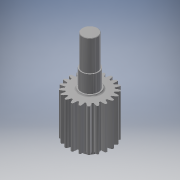
# Autodesk Inventor part: Spur Gear1
Saved by Autodesk Inventor 2018 (Build 220112000, 112)
## iProperties
Created: 2018-12-20
Part Number: Spur Gear1
Material: Steel
Document SubType Name: Modeling
Designer: Kristijan
Categories: <?xml version="1.0" encoding="UTF-16"?> <MemberInstance><Categories><FamilyTemplate><FamilyTemplateParameter ValueType="xs:double" Id="1" ObjectReferenceKey="da_z" ObjectType="kUserParameterObject"/><FamilyTemplateParameter ValueType="xs:double" Id="2" ObjectReferenceKey="da_b" ObjectType="kUserParameterObject"/><FamilyTemplateParameter ValueType="xs:double" Id="3" ObjectReferenceKey="da_beta" ObjectType="kUserParameterObject"/><FamilyTemplateParameter ValueType="xs:double" Id="4" ObjectReferenceKey="da_da" ObjectType="kUserParameterObject"/><FamilyTemplateParameter ValueType="xs:double" Id="5" ObjectReferenceKey="da_aw" ObjectType="kUserParameterObject"/><FamilyTemplateParameter ValueType="xs:string" Id="6" ObjectReferenceKey="EAIAABAAAACIAQAAAAAAAIAAAAAAAAAA" ObjectType="83910656" SubObjectId="SurfaceGeometry"/></FamilyTemplate><ParamToTemplateMap><ParamToTemplate CategoryParameter="//CategoryParameter[@InternalName='046C89C9-8512-4d59-83FE-43B91F4F132A']" TemplateParameter="1"/><ParamToTemplate CategoryParameter="//CategoryParameter[@InternalName='2552DF32-E462-4b46-AEBF-C6C7768E72AC']" TemplateParameter="2"/><ParamToTemplate CategoryParameter="//CategoryParameter[@InternalName='C9EE641D-15FC-4fae-A226-E94C4372FDD7']" TemplateParameter="3"/><ParamToTemplate><ParamToTemplate CategoryParameter="//CategoryParameter[@InternalName='00B6519A-459B-49c7-AD84-2E56D39A5744']" ConstantValue="0.000000"/></ParamToTemplate><ParamToTemplate><ParamToTemplate CategoryParameter="//CategoryParameter[@InternalName='04B31F0E-C7A6-4894-AA32-9629BEFACF47']" ConstantValue="1.000000"/></ParamToTemplate><ParamToTemplate><ParamToTemplate CategoryParameter="//CategoryParameter[@InternalName='43CBEC2E-7847-49e7-A936-2F7889FCB2D9']" ConstantValue="0.250000"/></ParamToTemplate><ParamToTemplate><ParamToTemplate CategoryParameter="//CategoryParameter[@InternalName='B1EFC894-105D-4ebd-86BF-FA20ED196853']" ConstantValue="0.350000"/></ParamToTemplate><ParamToTemplate><ParamToTemplate CategoryParameter="//CategoryParameter[@InternalName='51175063-3D10-4879-93E8-6246FE8B403D']" ConstantValue="2060000000.000000"/></ParamToTemplate><ParamToTemplate><ParamToTemplate CategoryParameter="//CategoryParameter[@InternalName='A3A52E27-4454-46a9-B0BD-C932399B70AF']" ConstantValue="0.300000"/></ParamToTemplate><ParamToTemplate><ParamToTemplate CategoryParameter="//CategoryParameter[@InternalName='91B76062-C214-41d9-B1B9-14D2AB99603D']" ConstantValue="0.500000"/></ParamToTemplate><ParamToTemplate><ParamToTemplate CategoryParameter="//CategoryParameter[@InternalName='374E806E-8B8A-4dda-A9AA-1039D6500AD2']" ConstantValue="2.000000"/></ParamToTemplate><ParamToTemplate><ParamToTemplate CategoryParameter="//CategoryParameter[@InternalName='2D373A89-B862-43d6-8D0B-0CBF12AB9F6C']" ConstantValue="0.349066"/></ParamToTemplate><ParamToTemplate CategoryParameter="//CategoryParameter[@InternalName='37777632-D6A2-4fac-9D53-DB8ACD95C989']" TemplateParameter="4"/><ParamToTemplate CategoryParameter="//CategoryParameter[@InternalName='FD1017F1-B727-4f7e-9707-0F86F1FF9423']" TemplateParameter="5"/><ParamToTemplate><ParamToTemplate CategoryParameter="//CategoryParameter[@InternalName='9E1B4470-B2D3-4ff1-B813-535BB4CDF51A']" ConstantValue="3520000.000000"/></ParamToTemplate><ParamToTemplate><ParamToTemplate CategoryParameter="//CategoryParameter[@InternalName='F8452263-BFF6-458c-9FB1-07C4B99E95CD']" ConstantValue="11400000.000000"/></ParamToTemplate><ParamToTemplate><ParamToTemplate CategoryParameter="//CategoryParameter[@InternalName='3E3BB259-FD49-497f-8171-6EBC954A3479']" ConstantValue="2.000000"/></ParamToTemplate><ParamToTemplate CategoryParameter="//CategoryParameter[@InternalName='27C3BAF2-7550-4e4b-AE2C-0DB134B7D9B7']" TemplateParameter="6"/></ParamToTemplateMap><Category DisplayName="Gear" InternalName="DC85795E-93AB-48d5-8EEE-5A27447B64BD" Mnemonic="Gear"><CategoryParameter DisplayName="z" InternalName="046C89C9-8512-4d59-83FE-43B91F4F132A" Mnemonic="z"/><CategoryParameter DisplayName="b" InternalName="2552DF32-E462-4b46-AEBF-C6C7768E72AC" Mnemonic="b"/><CategoryParameter DisplayName="||b|" InternalName="C9EE641D-15FC-4fae-A226-E94C4372FDD7" Mnemonic="beta"/><CategoryParameter DisplayName="x" InternalName="00B6519A-459B-49c7-AD84-2E56D39A5744" Mnemonic="x"/><CategoryParameter DisplayName="a*" InternalName="04B31F0E-C7A6-4894-AA32-9629BEFACF47" Mnemonic="a"/><CategoryParameter DisplayName="c*" InternalName="43CBEC2E-7847-49e7-A936-2F7889FCB2D9" Mnemonic="c"/><CategoryParameter DisplayName="r|.f|*" InternalName="B1EFC894-105D-4ebd-86BF-FA20ED196853" Mnemonic="rf"/><CategoryParameter DisplayName="E" InternalName="51175063-3D10-4879-93E8-6246FE8B403D" Mnemonic="E"/><CategoryParameter DisplayName="||m|" InternalName="A3A52E27-4454-46a9-B0BD-C932399B70AF" Mnemonic="mi"/><Category DisplayName="SpurGear" InternalName="26C5A22E-A91E-4dfd-A3B3-23CCAFAE1764" Mnemonic="SpurGear"><CategoryParameter DisplayName="m" InternalName="91B76062-C214-41d9-B1B9-14D2AB99603D" Mnemonic="m"/><CategoryParameter DisplayName="P" InternalName="374E806E-8B8A-4dda-A9AA-1039D6500AD2" Mnemonic="PP"/><CategoryParameter DisplayName="||a|" InternalName="2D373A89-B862-43d6-8D0B-0CBF12AB9F6C" Mnemonic="alpha"/><CategoryParameter DisplayName="d|.a|" InternalName="37777632-D6A2-4fac-9D53-DB8ACD95C989" Mnemonic="da"/><CategoryParameter DisplayName="a|.w|" InternalName="FD1017F1-B727-4f7e-9707-0F86F1FF9423" Mnemonic="aw"/><CategoryParameter DisplayName="||s||.Flim|" InternalName="9E1B4470-B2D3-4ff1-B813-535BB4CDF51A" Mnemonic="sFlim"/><CategoryParameter DisplayName="||s||.Hlim|" InternalName="F8452263-BFF6-458c-9FB1-07C4B99E95CD" Mnemonic="sHlim"/><CategoryParameter DisplayName="type" InternalName="3E3BB259-FD49-497f-8171-6EBC954A3479" Mnemonic="type"/><CategoryParameter DisplayName="PitchDiameter" InternalName="27C3BAF2-7550-4e4b-AE2C-0DB134B7D9B7" Mnemonic="IDS_PITCHDIAM"/></Category></Category></Categories></MemberInstance>
Density: 1 g/cm^3
Appearance: Steel
CustomPartVersion: 1
Author: Kristijan
Autodesk Inventor part; units mm, degrees
sketch "Sketch1" plane through (0, 0, 0) normal (0, 0, 1) x (1, 0, 0)
  circle A0 centre (0, 0) radius 57.5
  dimension "d0" = 115
  constraints: 1 centre point
  measures "d0" diameter of A0
extrude "Extrusion1" add sketch "Sketch1" along normal blind 110
ref_plane "Work Plane2" through (0, 0, 55) normal (0, 0, 1) x (1, 0, 0)
sketch "Sketch2" plane through (0, 0, 0) normal (0, 0, -1) x (-1, 0, 0)
  circle A0 centre (0, 0) radius 57.5 projected
  circle A1 centre (0, 0) radius 52.5
  dimension "d3" = 105
  constraints: 1 centre point, 1 coincident
  measures "d3" diameter of A1
surface extrude "Pitch Diameter" sketch "Sketch2" against normal through all shown no curves A1
ref_plane "Work Plane8" through (0, 0, 0) normal (0.9888308, 0.1490423, 0) x (0, 0, 1)
ref_plane "Work Plane9" through (0, 0, 0) normal (1, 0, 0) x (0, 1, 0)
spur gear teeth "Spur Gear" teeth 21 pitch diameter 105 tip diameter 115 root diameter 92.5 face width 110 start plane through (0, 0, 0) normal (0, 0, -1) x (-1, 0, 0)
sketch "Sketch3" plane through (0, 0, 110) normal (0, 0, 1) x (1, 0, 0)
  point P0 (0, 0)
sketch "Sketch4" plane through (0, 0, 0) normal (1, 0, 0) x (0, 1, 0)
  line L0 (0, 110) -> (29, 110)
  line L1 (25.4645, 113.5355) -> (22.5, 113.5355)
  line L2 (22.5, 113.5355) -> (22.5, 158.5355)
  line L3 (22.5, 158.5355) -> (20, 158.5355)
  line L4 (20, 158.5355) -> (20, 237.5355)
  line L5 (19, 238.5355) -> (0, 238.5355)
  line L6 (0, 238.5355) -> (0, 110)
  line L7 (19, 238.5355) -> (20, 237.5355)
  arc A0 (25.4645, 113.5355) -> (29, 110) centre (30.2941, 114.8296) ccw
  point P0 (0, 0)
  point P1 (20, 238.5355)
  point P2 (57.4598, 0)
  point P3 (34.1447, 0)
  dimension "d49" = 29
  dimension "d50" = 5
  dimension "d52" = 22.5
  dimension "d53" = 20
  dimension "d54" = 80
  dimension "d55" = 1
  dimension "d56" = 45
  dimension "d86" = 45
  constraints: 16 end point, 4 perpendicular, 2 horizontal, 2 point on circle, 2 point on line, 1 centre point
  measures "d49" distance of L0.start L0.end
  measures "d50" distance of L0.end L1.start
  measures "d52" distance between parallel lines of L6 L2
  measures "d53" distance between parallel lines of L6 L4
  measures "d54" distance of L3.end point (20, 238.536)
  measures "d55" distance of L5.start point (20, 238.536)
  measures "d56" angle of L5 L7
  measures "d86" distance of L1.end L2.end
revolve "Revolution1" add sketch "Sketch4" angle 360 about axis through (0, 0, 238.5355) along (0, 0, -1)
sketch "Sketch5" plane through (0, 0, 0) normal (1, 0, 0) x (0, 1, 0)
  line L0 (0, 0) -> (24, 0)
  line L1 (24, -5) -> (24, -5)
  line L2 (24, -5) -> (22.5, -5)
  line L3 (22.5, -5) -> (22.5, -24)
  line L4 (21.5, -25) -> (0, -25)
  line L5 (0, -25) -> (0, 0)
  line L6 (35.0562, 0) -> (46.2644, 0) projected
  line L7 (45.4437, 0) -> (45.4437, 110) construction
  line L8 (34.1447, 0) -> (37.5065, 0) construction
  line L9 (45.4437, 0) -> (29, 0) construction
  arc A0 (29, 0) -> (24, -5) centre (29, -5) ccw
  line L10 (22.5, -24) -> (21.5, -25)
  line L11 (24, 0) -> (29, 0)
  line L12 (24.6065, 0) -> (34.1447, 0) projected
  line L13 (0, -78) -> (0, 293) projected
  point P0 (22.5, -25)
  dimension "d73" = 5
  dimension "d74" = 22.5
  dimension "d75" = 20
  dimension "d76" = 1.5
  dimension "d77" = 1
  dimension "d78" = 45
  dimension "d79" = 25
  constraints: 18 end point, 5 perpendicular, 4 point on line, 3 tangent, 2 horizontal, 2 point on circle, 1 centre point, 1 collinear
  measures "d73" radius of A0
  measures "d74" distance of point (22.5, -25) L4.end
  measures "d75" distance of L2.end point (22.5, -25)
  measures "d76" distance of L1.end L2.end
  measures "d77" distance of L3.end point (22.5, -25)
  measures "d78" angle of L3 L10
  measures "d79" distance of L4.end L0.start
revolve "Revolution2" add sketch "Sketch5" angle 360 about axis through (0, 0, 0) along (0, 0, 1)
ref_plane "Work Plane11" through (0, 20, 198.0355) normal (0, 1, 0) x (-1, 0, 0)
sketch "Sketch6" plane through (0, 20, 198.0355) normal (0, 1, 0) x (-1, 0, 0)
  line L0 (20, 39.5) -> (20, -39.5) projected
  line L1 (-20, 39.5) -> (20, 39.5) projected
  line L2 (-20, -39.5) -> (20, -39.5) projected
  line L3 (-20, 39.5) -> (-20, -39.5) projected
  line L4 (-22.5, -39.5) -> (22.5, -39.5) projected
  line L5 (-22.5, -39.5) -> (22.5, -39.5) projected
  line L6 (-22.5, -84.5) -> (22.5, -84.5) projected
  line L7 (0, -266.5426) -> (0, 108.0071) projected
  line L8 (0, 30.5) -> (0, -29.5) construction
  line L9 (5, 30.5) -> (5, -29.5)
  line L10 (-5, -29.5) -> (-5, 30.5)
  arc A0 (5, 30.5) -> (-5, 30.5) centre (0, 30.5) ccw
  arc A1 (-5, -29.5) -> (5, -29.5) centre (0, -29.5) ccw
  point P0 (0, -198.0355)
  point P1 (0, 0.5)
  dimension "d81" = 10
  dimension "d84" = 10
  dimension "d87" = 70
  constraints: 8 end point, 4 point on circle, 4 tangent, 2 centre point, 2 point on line, 1 midpoint, 1 parallel
  measures "d81" distance between parallel lines of L10 L9
  measures "d84" distance from line of L2 L8.end
extrude "Extrusion2" cut sketch "Sketch6" against normal blind 5 contours A0 L9 A1 L7 | L7 A1 L10 A0
equation "\"d0\" = da_da"
equation "\"d1\" = da_b"
equation "\"d3\" = da_dw"
equation "\"d16\" = da_aw"
equation "\"d43\" = da_aw"
equation "\"d46\" = da_aw"
equation "\"da_da\" = 115"
equation "\"da_b\" = 110"
equation "\"da_dw\" = 105"
equation "\"da_aw\" = 262.5"
body "Solid1"
body "Srf1"
